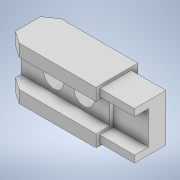
# Autodesk Inventor part: chodecsemafor
Saved by Autodesk Inventor 2020 (Build 240168000, 168)
## iProperties
Created: 2019-11-22
Part Number: chodecsemafor
Material: Všeobecné
Document SubType Name: Modeling
Designer: kotel
Density: 1 g/cm^3
Appearance: Výchozí
Author: kotel
Autodesk Inventor part; units mm, degrees
ref_plane "YZ Plane" through (0, 0, 0) normal (1, 0, 0) x (0, 1, 0)
ref_plane "XZ Plane" through (0, 0, 0) normal (0, 1, 0) x (-1, 0, 0)
ref_plane "XY Plane" through (0, 0, 0) normal (0, 0, 1) x (1, 0, 0)
sketch "Náčrt1" plane through (0, 0, 0) normal (0, 1, 0) x (-1, 0, 0)
  line L0 (0, 0) -> (50, 0)
  line L1 (50, 0) -> (66.0697, -19.1511)
  line L2 (50, 0) -> (75, 0) construction
  line L3 (66.0697, -19.1511) -> (58.4092, -25.579)
  line L4 (0, -12) -> (0, 0)
  line L5 (58.6554, -25.3724) -> (47.4347, -12)
  line L6 (47.4347, -12) -> (0, -12)
  dimension "d0" = 50
  dimension "d2" = 25
  dimension "d3" = 50
  dimension "d4" = 10
  dimension "d5" = 12
  constraints: 14 end point, 3 horizontal, 2 perpendicular, 1 equal length, 1 parallel, 1 point on line
  measures "d0" distance of L0.start L0.end
  measures "d2" distance of L0.end L1.end
  measures "d3" angle of L1 L2
  measures "d4" distance of L1.end L3.end
  measures "d5" distance of L4.start L0.start
extrude "Vysunutí1" add sketch "Náčrt1" along normal blind 15
sketch "Náčrt11" plane through (0, 0, 0) normal (1, 0, 0) x (0, 0, -1)
  line L0 (0, 0) -> (0, 15) projected
  line L1 (0, 7.5) -> (12, 7.5)
  line L2 (12, 0) -> (12, 15) projected
  line L3 (0, 3.5) -> (4, 3.5)
  line L4 (4, 3.5) -> (4, 11.5)
  line L5 (4, 11.5) -> (0, 11.5)
  line L6 (0, 11.5) -> (0, 3.5)
  point P0 (0, 7.5)
  point P1 (0, 11.5)
  dimension "d64" = 4
  dimension "d65" = 8
  constraints: 10 end point, 3 midpoint, 2 parallel, 1 horizontal, 1 perpendicular, 1 point on line, 1 other
  measures "d64" distance of L5.end L4.end
  measures "d65" distance of L4.end L3.end
extrude "Vysunutí10" cut sketch "Náčrt11" against normal through all
sketch "Náčrt21" plane through (-66.0697, 0, -19.1511) normal (-0.6427876, 0, -0.7660444) x (-0.7660444, 0, 0.6427876)
  line L0 (0, 0) -> (0, 15) projected
  line L1 (0, 3.5) -> (-4, 3.5)
  line L2 (-4, 3.5) -> (-4, 11.5)
  line L3 (-4, 11.5) -> (0, 11.5)
  line L4 (0, 11.5) -> (0, 3.5)
  point P0 (-38.3022, 0)
  point P1 (0, 7.5)
  point P2 (0, 11.5)
  dimension "d68" = 4
  dimension "d69" = 8
  constraints: 8 end point, 3 perpendicular, 2 parallel, 1 horizontal, 1 midpoint, 1 point on line, 1 other
  measures "d68" distance of L2.end L3.end
  measures "d69" distance of L1.end L2.end
extrude "Vysunutí11" cut sketch "Náčrt21" against normal through all
sketch "Náčrt30" plane through (0, 0, -12) normal (0, 0, -1) x (-1, 0, 0)
  point P0 (0, 0)
sketch "Náčrt31" plane through (0, 0, 0) normal (1, 0, 0) x (0, 0, -1)
  point P0 (0, 0)
sketch "Náčrt32" plane through (0, 0, 0) normal (0, -1, 0) x (1, 0, 0)
  line L0 (-47.4347, -12) -> (-58.6554, -25.3724) projected
  line L1 (-47.4347, -12) -> (-47.4347, 0)
  line L2 (-47.4347, -12) -> (-58.6554, -25.3724)
  line L3 (-58.6554, -25.3724) -> (-66.0697, -19.1511) projected
  line L4 (-66.0697, -19.1511) -> (-50, 0)
  line L5 (-50, 0) -> (-47.4347, 0)
  line L6 (-50, 0) -> (0, 0) projected
  point P0 (-47.4347, 0)
  constraints: 8 end point, 1 collinear, 1 parallel, 1 perpendicular, 1 vertical
extrude "Vysunutí16" add sketch "Náčrt32" against normal through all
sketch "Náčrt33" plane through (0, 0, 0) normal (0, -1, 0) x (1, 0, 0)
  line L0 (-47.4347, -12) -> (-58.6554, -25.3724) projected
  line L1 (-47.4347, -4) -> (-47.4347, 0) projected
  line L2 (-47.4347, -12) -> (-47.4347, 0)
  line L3 (-66.0697, -19.1511) -> (-50, 0) projected
  line L4 (-47.4347, 0) -> (-50, 0)
  line L5 (-50, 0) -> (-66.0697, -19.1511)
  line L6 (-50, 0) -> (0, 0) projected
  line L7 (-66.0697, -19.1511) -> (-50, 0) projected
  line L8 (-58.6554, -25.3724) -> (-66.0697, -19.1511) projected
  line L9 (-47.4347, -12) -> (-58.6554, -25.3724) projected
  line L10 (0, -12) -> (-47.4347, -12) projected
  line L11 (0, 0) -> (0, -12) projected
  line L12 (-58.6554, -25.3724) -> (-66.0697, -19.1511) projected
  line L13 (-66.0697, -19.1511) -> (-58.6554, -25.3724)
  line L14 (-58.6554, -25.3724) -> (-47.4347, -12)
  constraints: 10 end point, 3 collinear, 1 perpendicular, 1 vertical
extrude "Vysunutí17" cut sketch "Náčrt33" against normal through all contours L0 L8 L3 L4 L1 L2
sketch "Náčrt34" plane through (0, 0, 0) normal (0, -1, 0) x (1, 0, 0)
  line L0 (-47.4347, 0) -> (-47.4347, -12) projected
  line L1 (-47.4347, 0) -> (-47.4347, -12) projected
  line L2 (0, -12) -> (-47.4347, -12) projected
  line L3 (0, 0) -> (0, -12) projected
  line L4 (-47.4347, 0) -> (0, 0) projected
  line L5 (0, -12) -> (-47.4347, -12) projected
  line L6 (-44, -12) -> (-47.4347, -9.595)
  line L7 (-44, -12) -> (-39.807, -12) construction
  line L8 (-47.4347, -9.595) -> (-47.4347, -12)
  line L9 (-44, -12) -> (-47.4347, -12)
  line L10 (0, 0) -> (-47.4347, 0) projected
  line L11 (-44, 0) -> (-47.0563, -2.14)
  line L12 (-44, 0) -> (-40.269, 0) construction
  line L13 (-47.0563, -2.14) -> (-47.4347, -2.405)
  line L14 (-47.4347, -2.405) -> (-47.4347, 0)
  line L15 (-44, 0) -> (-47.4347, 0)
  dimension "d99" = 145
  dimension "d100" = 145
  constraints: 18 end point, 5 point on line, 2 collinear, 2 equal length, 2 horizontal, 2 perpendicular
  measures "d99" angle of L7 L6
  measures "d100" angle of L11 L12
extrude "Vysunutí18" cut sketch "Náčrt34" against normal through all contours L4 L11 L13 L0 | L6 L2 L0
sketch "Náčrt39" plane through (0, 0, 0) normal (1, 0, 0) x (0, 0, -1)
  line L0 (0, 11.5) -> (0, 15) projected
  line L1 (12, 0) -> (12, 15) projected
  line L2 (0, 0) -> (0, 3.5) projected
  line L3 (1, 0.75) -> (10, 0.75)
  line L4 (10, 14.25) -> (1, 14.25)
  line L5 (1, 14.25) -> (1, 12.2503)
  line L6 (4, 4.7) -> (4, 10.3) projected
  line L7 (5, 12.2503) -> (1, 12.2503)
  line L8 (1, 0.75) -> (1, 2.7496)
  line L9 (1, 2.7496) -> (5, 2.7496)
  line L10 (5, 2.7496) -> (5, 12.2503)
  line L11 (10, 0.75) -> (10, 14.25)
  line L12 (4, 7.5) -> (12, 7.5)
  line L13 (12, 9.95) -> (12, 5.05) projected
  point P0 (1, 1.7498)
  point P1 (5, 7.5)
  point P2 (1, 13.2502)
  point P3 (10, 7.5)
  point P4 (5.5, 0.75)
  dimension "d119" = 13.5
  constraints: 18 end point, 7 midpoint, 3 vertical, 2 horizontal, 1 parallel, 5 other
  measures "d119" distance of L3.end L4.start
extrude "Vysunutí22" add sketch "Náčrt39" along normal blind 10
sketch "Náčrt40" plane through (0, 0, 0) normal (0, -1, 0) x (1, 0, 0)
  line L0 (-47.4347, -2.405) -> (-47.4347, -9.595) projected
  line L1 (-47.4347, -6) -> (0, -6)
  line L2 (-44, 0) -> (-47.4347, -2.405) projected
  line L3 (-47.4347, -2.405) -> (-47.4347, -9.595) projected
  line L4 (-47.4347, -9.595) -> (-44, -12) projected
  line L5 (0, -12) -> (-44, -12) projected
  line L6 (0, 0) -> (0, -12) projected
  line L7 (-44, 0) -> (0, 0) projected
  line L8 (-27.885, -6) -> (-22.985, -6) projected
  line L9 (-25.435, -6) -> (-25.435, 0)
  line L10 (-25.435, -6) -> (-25.435, -12)
  dimension "d124" = 47.4347
  constraints: 6 end point, 3 point on line, 2 midpoint, 1 horizontal, 1 perpendicular
  measures "d124" distance of L1.start L1.end
extrude "Vysunutí24" cut sketch "Náčrt40" against normal through all contours L2 L7 L9 L1 L0 | L1 L10 L5 L4 L0
sketch "Náčrt41" plane through (0, 15, 0) normal (0, 1, 0) x (1, 0, 0)
  line L0 (-25.435, 0) -> (0, 0) projected
  line L1 (-25.435, 0) -> (-22, 0)
  line L2 (-22, 0) -> (-25.435, 2.4052)
  line L3 (-25.435, 12) -> (-25.435, 0) projected
  line L4 (-25.435, 2.4052) -> (-25.435, 0)
  line L5 (-22, 0) -> (-25.435, 0)
  line L6 (0, 12) -> (-25.435, 12) projected
  line L7 (-22, 12) -> (-17.9846, 12) construction
  line L8 (-25.435, 9.6038) -> (-21.9829, 12)
  line L9 (-25.435, 9.6038) -> (-25.435, 12)
  line L10 (-21.9829, 12) -> (-25.435, 12)
  dimension "d127" = 3.435
  dimension "d128" = 35
  constraints: 16 end point, 5 point on line, 2 collinear, 1 horizontal, 1 perpendicular, 1 vertical
  measures "d127" distance of L0.start L1.end
  measures "d128" angle of L2 L1
extrude "Vysunutí25" cut sketch "Náčrt41" against normal through all
sketch "Náčrt42" plane through (0, 3.5, -4) normal (0, 0, 1) x (1, 0, 0)
  line L0 (-25.435, 8) -> (-25.435, 0) projected
  line L1 (-25.435, 4) -> (0, 4)
  line L2 (0, -3.5) -> (0, 11.5) projected
  line L3 (-21.9829, -3.5) -> (-21.9829, 11.5) projected
  line L4 (-21.9829, 4) -> (-16.0829, 4)
  circle A0 centre (-16.0829, 4) radius 2.9
  line L5 (-13.1829, 4) -> (-10.1829, 4)
  circle A1 centre (-7.3829, 4) radius 2.9
  line L6 (-10.2829, 7.4092) -> (-10.2829, 0.965)
  dimension "d133" = 5.8
  dimension "d132" = 5.9
  dimension "d134" = 3
  dimension "d136" = 5.8
  constraints: 8 end point, 4 point on line, 3 midpoint, 1 centre point, 1 coincident, 1 horizontal alignment, 1 perpendicular, 1 tangent, 1 vertical, 2 other
  measures "d132" distance of L4.start L4.end
  measures "d134" distance of L5.start L5.end
  measures "d136" diameter of A1
extrude "Vysunutí26" cut sketch "Náčrt42" against normal through all
